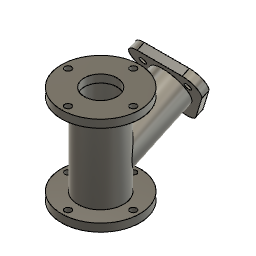
1.4 Part (Autodesk Fusion 360 design; units mm, degrees)
Autodesk Fusion 360 part; units mm, degrees
sketch "Sketch1" plane through (0, 0, 0) normal (0, 1, 0) x (1, 0, 0)
  circle A0 centre (0, 0) radius 35
  circle A1 centre (0, 0) radius 25
  dimension "d1" = 70
  dimension "d9" = 50
  constraint coincident A0.centre A1.centre
  constraint concentric A0 A1
  measures "d1" diameter of A0
  measures "d9" diameter of A1
extrude "Extrude2" add sketch "Sketch1" along normal blind 126 makes body 1
sketch "Sketch4" plane through (0, 0, 0) normal (1, 0, 0) x (0, 0, -1)
  line L0 (0, 38) -> (108.7569, 88.7142) construction
  line L1 (35, 0) -> (-35, 0)
  line L2 (0, 0) -> (109.8394, 0) construction
  dimension "d12" = 25
  dimension "d13" = 38
  dimension "d14" = 120
  constraint coincident L2.start origin
  constraint horizontal L2
  constraint vertical L0.start L2.start
  measures "d12" angle of L0 L2
  measures "d13" vertical distance of L0.start L2.start
  measures "d14" distance of L0.start L0.end
ref_plane "WorkPlane2" through (0, 88.1385, -107.5224) normal (0, 0.422618, -0.906308) x (-1, 0, 0)
sketch "Sketch5" plane through (0, 88.1385, -107.5224) normal (0, 0.422618, -0.906308) x (-1, 0, 0)
  circle A0 centre (0, 0) radius 30
  circle A1 centre (0, 0) radius 18
  dimension "d16" = 60
  dimension "d17" = 36
  constraint coincident A0.centre A1.centre
  constraint concentric A0 A1
  measures "d16" diameter of A0
  measures "d17" diameter of A1
extrude "Extrude3" add sketch "Sketch5" along normal up to surface separate body end surface at (34.9565, 42, 1.7446) on bodies 1 makes body 2
sketch "Sketch6" plane through (0, 56.9256, -122.0773) normal (0, 0.422618, -0.906308) x (-1, 0, 0)
  circle A0 centre (0, 34.4397) radius 18
  circle A1 centre (0, 34.4397) radius 30
  line L0 (0, 34.4397) -> (0, -5.5603) construction
  circle A2 centre (0, -5.5603) radius 5.4
  circle A3 centre (34.4964, 54.6882) radius 5.4
  circle A4 centre (-34.4964, 54.6881) radius 5.4
  line L1 (-34.4964, 74.6881) -> (34.5598, 74.6881)
  line L2 (-51.8527, 44.7504) -> (-17.3563, -15.498)
  line L3 (51.8721, 44.7845) -> (17.3563, -15.498)
  arc A5 (-34.4964, 74.6881) -> (-51.8527, 44.7504) centre (-34.4964, 54.6881) ccw
  arc A6 (51.8721, 44.7845) -> (34.5598, 74.6881) centre (34.4964, 54.6882) ccw
  circle A7 centre (0, -5.5603) radius 20
  circle A8 centre (0, 34.4397) radius 20
  point P0 (0, 34.4397)
  dimension "d23" = 10.8
  dimension "d26" = 40
  constraint horizontal L1
  constraint tangent L1 A5
  constraint tangent L2 A5
  constraint concentric A2 A7
  constraint coincident P0 A0.centre
  constraint tangent A5 A8
  constraint tangent A7 A8
  constraint tangent L2 A7
  constraint coincident A7 L2.end
  constraint coincident A4.centre A5.centre
  constraint coincident A3.centre A6.centre
  measures "d23" diameter of A2
  measures "d26" diameter of A7
extrude "Extrude4" add sketch "Sketch6" along normal blind 12 separate body contours A1 A7 | A1 L1 L2 L3 A5 A6 A7 | A1 A7 | A1 A7 makes body 3
extrude "Extrude5" add 1 faces at (-25.8213, 85.9773, -108.5302) along direction (0, 0.422618, -0.906308) blind 4 on bodies 2 bodies 1 2 3
sketch "Sketch7" plane through (0, 126, 0) normal (0, 1, 0) x (-1, 0, 0)
  circle A0 centre (0, 0) radius 25
  circle A1 centre (0, 0) radius 35
  circle A2 centre (0, 0) radius 60
  circle A3 centre (0, 0) radius 50 construction
  circle A4 centre (0, -50) radius 5
  circle A5 centre (50, 0) radius 5
  circle A6 centre (0, 50) radius 5
  circle A7 centre (-50, 0) radius 5
  dimension "d32" = 120
  dimension "d33" = 100
  dimension "d34" = 10
  dimension "d36" = 360
  constraint concentric A0 A2
  constraint concentric A2 A3
  constraint coincident A3 A4.centre
  measures "d32" diameter of A2
  measures "d33" diameter of A3
  measures "d34" diameter of A4
extrude "Extrude6" add sketch "Sketch7" along normal blind 12 contours A1 | A2 bodies 2 makes body 4
ref_plane "WorkPlane3" through (0, 63, 0) normal (0, -1, 0) x (1, 0, 0)
mirror "Mirror1" about plane through (0, 63, 0) normal (0, -1, 0) of "Extrude6" makes body 5
ref_plane "WorkPlane5" through (0, 98.9711, -130.7529) normal (0, 0.422618, -0.906308) x (-1, 0, 0)
move_body "Move1" bodies 1 2 4 5 to x (1, 0, 0) y (0, 1, 0) z (0, 0, 1) at (0, 13.2887, 0)
